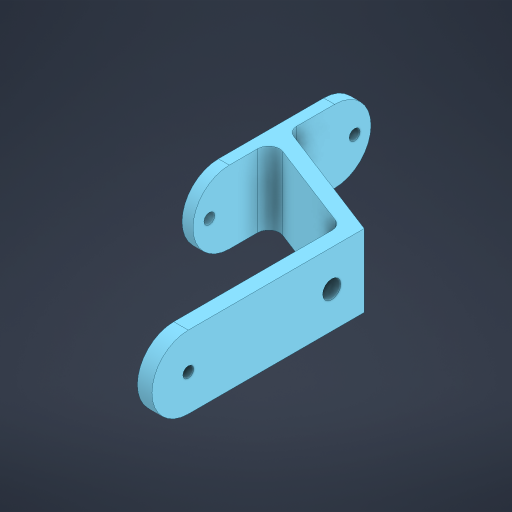
# Autodesk Inventor part: acople_3
Saved by Autodesk Inventor 2023.1 (Build 271208000, 208)
## iProperties
Created: 2022-10-29
Part Number: acople_3
Material: Generic
Document SubType Name: Modeling
Designer: amtat
Density: 1 g/cm^3
Appearance: Default
Author: amtat
Autodesk Inventor part; units mm, degrees
ref_plane "YZ Plane" through (0, 0, 0) normal (1, 0, 0) x (0, 1, 0)
ref_plane "XZ Plane" through (0, 0, 0) normal (0, 1, 0) x (-1, 0, 0)
ref_plane "XY Plane" through (0, 0, 0) normal (0, 0, 1) x (1, 0, 0)
sketch "Sketch1" plane through (0, 0, 0) normal (1, 0, 0) x (0, 1, 0)
  circle A0 centre (0, 0) radius 1.5
  line L0 (0, 0) -> (0, -40)
  circle A1 centre (0, -40) radius 1.5
  line L1 (0, 1.5) -> (0, 4.5)
  line L2 (0, -41.5) -> (0, -44.5)
  line L3 (0, -44.5) -> (0, -34.5)
  line L4 (0, 4.5) -> (0, -5.5)
  arc A2 (10, -5.5) -> (0, -15.5) centre (0, -5.5) ccw
  arc A3 (0, -24.5) -> (10, -34.5) centre (0, -34.5) ccw
  line L5 (10, -5.5) -> (10, -34.5)
  line L6 (-10, -5.5) -> (-10, -34.5)
  dimension "d0" = 3
  dimension "d2" = 3
  dimension "d1" = 40
  dimension "d3" = 3
  dimension "d4" = 3
  dimension "d5" = 10
  dimension "d6" = 10
  constraints: 14 end point, 8 point on circle, 4 coincident, 4 point on line, 3 vertical, 2 centre point, 2 tangent, 2 vertical alignment, 4 other
  measures "d1" distance of L0.start L0.end
  measures "d3" distance of L1.start L1.end
  measures "d4" distance of L2.start L2.end
  measures "d5" distance of L2.end L3.end
  measures "d6" distance of L1.end L4.end
extrude "Extrusion1" add sketch "Sketch1" along normal blind 3 contours A0 L1 A2 L5 A3 L2 A1 L0 | A0 L0 A2 L1 | A2 L0 A3 L6 | A3 L0 A1 L2
sketch "Sketch2" plane through (0, -10, -34.5) normal (0, -1, 0) x (1, 0, 0)
  line L0 (0, 29) -> (0, 0) projected
  line L1 (0, 0) -> (3, 0) projected
  line L2 (3, 29) -> (3, 0) projected
  line L3 (0, 29) -> (3, 29) projected
  line L4 (3, 29) -> (35.7, 29)
  line L5 (35.7, 29) -> (39.7, 29)
  line L6 (35.7, 29) -> (35.7, 89)
  line L7 (35.7, 89) -> (39.7, 89)
  line L8 (39.7, 89) -> (39.7, 29)
  point P0 (0, 34.5)
  dimension "d9" = 32.7
  dimension "d10" = 4
  dimension "d11" = 60
  constraints: 10 end point, 2 horizontal, 2 perpendicular, 1 vertical
  measures "d9" distance of L2.start L4.end
  measures "d10" distance of L4.end L5.end
  measures "d11" distance of L4.end L6.end
extrude "Extrusion2" add sketch "Sketch2" against normal blind 20 contours L6 L7 L8 L5
sketch "Sketch3" plane through (35.7, -10, -5.5) normal (-1, 0, 0) x (0, 0, 1)
  circle A0 centre (5.5, 10) radius 1.5 projected
  line L0 (5.5, 10) -> (12, 10)
  line L1 (12, 10) -> (32, 10)
  line L2 (32, 10) -> (45, 10)
  circle A1 centre (45, 10) radius 13
  dimension "d14" = 6.5
  dimension "d15" = 20
  dimension "d16" = 13
  constraints: 6 end point, 3 horizontal, 1 coincident, 1 horizontal alignment, 2 other
  measures "d14" distance of L0.start L0.end
  measures "d15" distance of L0.end L1.end
  measures "d16" distance of L1.end L2.end
extrude "Extrusion3" add sketch "Sketch3" against normal blind 4 contours A1
sketch "Sketch4" plane through (35.7, -10, 54.5) normal (-1, 0, 0) x (0, 0, 1)
  line L0 (0, 0) -> (-6.6934, 0) projected
  line L1 (0, 0) -> (0, 20) projected
  line L2 (-6.6934, 20) -> (0, 20) projected
  arc A0 (-6.6934, 20) -> (-23.3066, 20) centre (-15, 10) ccw projected
  line L3 (-60, 20) -> (-23.3066, 20) projected
  line L4 (-60, 0) -> (-60, 20) projected
  line L5 (-23.3066, 0) -> (-60, 0) projected
  arc A1 (-23.3066, 0) -> (-6.6934, 0) centre (-15, 10) ccw projected
  circle A2 centre (-15, 10) radius 13
  line L6 (-15, 10) -> (-25, 10)
  line L7 (-15, 10) -> (-15, 20)
  circle A3 centre (-25, 10) radius 0.5
  circle A4 centre (-15, 20) radius 0.5
  circle A5 centre (-5, 10) radius 0.5
  circle A6 centre (-15, 0) radius 0.5
  point P0 (-54.5, 10)
  dimension "d19" = 10
  dimension "d20" = 10
  dimension "d21" = 1
  dimension "d22" = 1
  constraints: 5 centre point, 4 end point, 3 coincident, 2 symmetric about line, 1 horizontal, 1 vertical, 2 other
  measures "d19" distance of L6.start L6.end
  measures "d20" distance of L6.start L7.end
  measures "d21" diameter of A3
  measures "d22" diameter of A4
extrude "Extrusion4" cut sketch "Sketch4" against normal blind 4 contours L0 A2 L2 L1 | A3 | A4 | A5 | A6
sketch "Sketch7" plane through (35.7, -10, -5.5) normal (-1, 0, 0) x (0, 0, 1)
  arc A0 (36.6934, 0) -> (36.6934, 20) centre (45, 10) ccw projected
  line L0 (0, 20) -> (36.6934, 20) projected
  line L1 (0, 0) -> (0, 20) projected
  line L2 (36.6934, 0) -> (0, 0) projected
  circle A1 centre (35, 10) radius 0.5 projected
  circle A2 centre (45, 0) radius 0.5 projected
  circle A3 centre (45, 20) radius 0.5 projected
  circle A4 centre (55, 10) radius 0.5 projected
  point P0 (5.5, 10)
extrude "Extrusion7" add sketch "Sketch7" along normal blind 3
sketch "Sketch8" plane through (39.7, -10, -5.5) normal (1, 0, 0) x (0, 0, -1)
  arc A0 (-36.6934, 20) -> (-36.6934, 0) centre (-45, 10) ccw projected
  line L0 (0, 0) -> (-36.6934, 0) projected
  line L1 (0, 0) -> (0, 20) projected
  line L2 (-36.6934, 20) -> (0, 20) projected
  circle A1 centre (-55, 10) radius 0.5 projected
  circle A2 centre (-45, 20) radius 0.5 projected
  circle A3 centre (-45, 0) radius 0.5 projected
  circle A4 centre (-35, 10) radius 0.5 projected
  point P0 (-5.5, 10)
extrude "Extrusion8" cut sketch "Sketch8" against normal blind 3
sketch "Sketch10" plane through (0, -10, -34.5) normal (0, -1, 0) x (1, 0, 0)
  line L0 (0, 29) -> (0, 0) projected
  line L1 (0, 0) -> (3, 0) projected
  line L2 (3, 29) -> (3, 0) projected
  line L3 (0, 29) -> (3, 29) projected
  line L4 (32.7, 29) -> (3, 12.5) projected
  line L5 (3, 12.5) -> (36.7, 31.2222)
  point P0 (0, 34.5)
  constraints: 2 end point, 1 collinear
extrude "Extrusion10" [suppressed]
sketch "Sketch12" plane through (32.7, -10, -5.5) normal (0, 0, -1) x (-1, 0, 0)
  line L0 (-4, 20) -> (-4, 0) projected
  line L1 (0, 0) -> (-4, 0) projected
  line L2 (0, 20) -> (0, 0) projected
  line L3 (-4, 20) -> (0, 20) projected
  point P0 (32.7, 10)
extrude "Extrusion12" add sketch "Sketch12" along normal blind 5
sketch "Sketch13" plane through (0, 10, -5.5) normal (0, 1, 0) x (1, 0, 0)
  line L0 (0, 29) -> (0, 0) projected
  line L1 (0, 0) -> (3, 0) projected
  line L2 (3, 29) -> (3, 0) projected
  line L3 (0, 29) -> (3, 29) projected
  line L4 (0, 0) -> (3, 0) projected
  line L5 (3, 0) -> (3, 14.5)
  line L6 (3, 29) -> (3, 0) projected
  line L7 (3, 14.5) -> (3, 16.5)
  line L8 (32.7, -36.6934) -> (32.7, 5) projected
  line L9 (3, 16.5) -> (32.7, 5)
  line L10 (10.3918, 13.6379) -> (8.9475, 9.9077)
  line L11 (25.3699, 7.8382) -> (23.9256, 4.1081)
  line L12 (8.9475, 9.9077) -> (32.7, 0.7106)
  line L13 (23.9256, 4.1081) -> (3, 12.2106)
  point P0 (0, -5.5)
  point P1 (3, 12.2106)
  dimension "d55" = 14.5
  dimension "d56" = 2
  dimension "d57" = 4
  dimension "d58" = 4
  constraints: 14 end point, 6 point on line, 3 perpendicular, 1 midpoint
  measures "d55" distance of L1.end L5.end
  measures "d56" distance of L5.end L7.end
  measures "d57" distance of L10.start L10.end
  measures "d58" distance of L11.start L11.end
extrude "Extrusion13" add sketch "Sketch13" against normal blind 20 contours L9 L10 L13 L2 | L9 L11 L12 L10 | L9 L8 L12 L11
sketch "Sketch14" plane through (36.7, -10, -5.5) normal (1, 0, 0) x (0, 0, -1)
  circle A0 centre (-5.5, 10) radius 1.5 projected
  circle A1 centre (-5.5, 10) radius 2.5
  dimension "d61" = 5
  constraints: 1 centre point, 1 coincident
  measures "d61" diameter of A1
extrude "Extrusion14" cut sketch "Sketch14" against normal blind 5 contours A0 | A1
sketch "Sketch15" plane through (0, 10, -5.5) normal (0, 1, 0) x (1, 0, 0)
  line L0 (0, 29) -> (0, 0) projected
  line L1 (0, 0) -> (3, 0) projected
  line L2 (3, 12.2106) -> (3, 0) projected
  line L3 (3, 12.2106) -> (32.7, 0.7106) projected
  line L4 (32.7, -36.6934) -> (32.7, 0.7106) projected
  line L5 (32.7, -36.6934) -> (36.7, -36.6934) projected
  line L6 (36.7, -36.6934) -> (36.7, 5) projected
  line L7 (32.7, 5) -> (36.7, 5) projected
  line L8 (32.7, 5) -> (3, 16.5) projected
  line L9 (3, 29) -> (3, 16.5) projected
  line L10 (0, 29) -> (3, 29) projected
  line L11 (32.7, 5) -> (3, 16.5) projected
  line L12 (3, 16.5) -> (36.7, 3.4512)
  point P0 (0, -5.5)
  constraints: 2 end point, 2 point on line
extrude "Extrusion15" cut sketch "Sketch15" against normal through all contours L7 L6 L12
fillet "Fillet3" radius 3 3 edges at (3, 0, -17.7106) (32.7, 0, -6.2106) (3, 0, -22)
sketch "Sketch16" plane through (36.7, -10, -5.5) normal (1, 0, 0) x (0, 0, -1)
  circle A0 centre (-45, 20) radius 0.5 projected
  circle A1 centre (-35, 10) radius 0.5 projected
  circle A2 centre (-45, 0) radius 0.5 projected
  circle A3 centre (-55, 10) radius 0.5 projected
  point P0 (-5.5, 10)
extrude "Extrusion16" add sketch "Sketch16" against normal blind 4
sketch "Sketch17" plane through (36.7, -10, -5.5) normal (1, 0, 0) x (0, 0, -1)
  line L0 (3.4512, 0) -> (3.4512, 20) projected
  line L1 (-36.6934, 20) -> (3.4512, 20) projected
  arc A0 (-36.6934, 20) -> (-36.6934, 0) centre (-45, 10) ccw projected
  line L2 (3.4512, 0) -> (-36.6934, 0) projected
  circle A1 centre (-5.5, 10) radius 2.5 projected
  line L3 (-36.6934, 20) -> (3.4512, 20) projected
  line L4 (-36.6934, 20) -> (-53.3066, 20)
  arc A2 (-36.6934, 20) -> (-36.6934, 0) centre (-45, 10) ccw projected
  line L5 (-36.6934, 0) -> (-53.3066, 0)
  circle A3 centre (-45, 10) radius 1.5
  dimension "d69" = 3
  constraints: 4 end point, 2 point on circle, 1 centre point, 1 coincident, 1 horizontal, 1 parallel
  measures "d69" diameter of A3
extrude "Extrusion17" cut sketch "Sketch17" against normal blind 4 contours A0 L5 | L4 A0 | A3
sketch "Sketch18" plane through (36.7, -10, -5.5) normal (1, 0, 0) x (0, 0, -1)
  line L0 (-53.3066, 0) -> (3.4512, 0) projected
  line L1 (3.4512, 0) -> (3.4512, 20) projected
  line L2 (3.4512, 20) -> (-53.3066, 20) projected
  arc A0 (-53.3066, 20) -> (-53.3066, 0) centre (-45, 10) ccw projected
  circle A1 centre (-45, 10) radius 1.5 projected
  circle A2 centre (-5.5, 10) radius 2.5 projected
  circle A3 centre (-45, 10) radius 1.5 projected
  circle A4 centre (-45, 10) radius 10
  point P0 (-45, 0)
  point P1 (-45, 20)
  constraints: 1 centre point, 1 coincident, 1 tangent
extrude "Extrusion18" cut sketch "Sketch18" against normal blind 4 contours A0 L2 A4 L0
body "Solid1"
